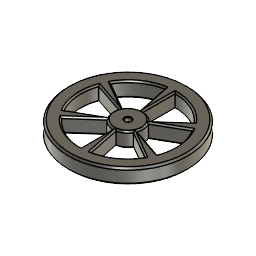
main_build (Autodesk Fusion 360 archive; units mm, degrees)
design "80x10 wheel"
Autodesk Fusion 360 part; units mm, degrees
sketch "Sketch1" plane through (0, 0, 0) normal (0, 0, 1) x (1, 0, 0)
  circle A0 centre (0, 0) radius 40
  dimension "d1" = 80
  constraint coincident A0.centre origin
  measures "d1" diameter of A0
extrude "Extrude1" add sketch "Sketch1" along normal blind 10
chamfer "Chamfer1" distance 1.2 angle 45 2 edges at (-37.2931, -14.4646, 10) (-37.2931, -14.4646, 0)
sketch "Sketch2" plane through (0, 0, 10) normal (0, 0, 1) x (-1, 0, 0)
  circle A0 centre (0, 0) radius 38.8
  circle A1 centre (0, 0) radius 1.5
  dimension "d5" = 3
  constraint coincident A0.centre A1.centre
  measures "d5" diameter of A1
extrude "Extrude2" cut sketch "Sketch2" against normal blind 25 contours A1
sketch "Sketch3" plane through (0, 0, 10) normal (0, 0, 1) x (-1, 0, 0)
  circle A0 centre (0, 0) radius 1.5
  circle A1 centre (0, 0) radius 38.8
  circle A2 centre (0, 0) radius 31.5
  circle A3 centre (0, 0) radius 10
  line L0 (0, -10) -> (0, -31.5)
  line L1 (-7.6037, -6.4949) -> (-23.6999, -20.75)
  dimension "d8" = 63
  dimension "d9" = 20
  constraint coincident A0.centre A1.centre
  constraint coincident A3 L0.start
  constraint coincident A2 L0.end
  constraint vertical L0
  constraint coincident A3 L1.start
  constraint coincident A2 L1.end
  measures "d8" diameter of A2
  measures "d9" diameter of A3
extrude "Extrude3" cut sketch "Sketch3" against normal blind 25 contours A2 A3 L0 L1 picked at (-16.9397, -17.3876)
chamfer "Chamfer2" distance 1 angle 45 6 edges at (13.012, 28.6869, 10) (15.6518, 13.6224, 10) (15.6518, 13.6224, 0) (0, 20.75, 10) (13.012, 28.6869, 0) (0, 20.75, 0)
pattern_circular "C-Pattern1" count 6 over 360 about axis through (0, 0, 1.75) along (0, 0, 1) of "Extrude3", "Chamfer2"
chamfer "Chamfer3" distance 1 angle 45 2 edges at (9.3233, 3.6162, 10) (7.7933, -6.2661, 0)
move_face "OffsetFaces1" offset -0.5 1 faces at (-1.4925, 0.1494, 6.6667)
chamfer "Chamfer4" distance 0.4 angle 45 1 edges at (1.8647, 0.7232, 0)
chamfer "Chamfer5" distance 0.4 angle 45 1 edges at (1.8647, -0.7232, 10)

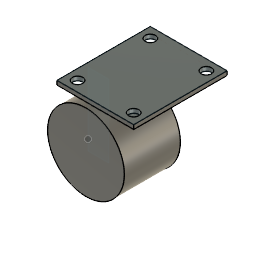
design "trolley_wheel"
Autodesk Fusion 360 part; units mm, degrees
sketch "Sketch1" plane through (0, 0, 0) normal (0, 0, 1) x (1, 0, 0)
  line L0 (0, 0) -> (37, 0)
  line L1 (37, 0) -> (37, 45)
  line L2 (37, 45) -> (0, 45)
  line L3 (0, 45) -> (0, 0)
  dimension "d1" = 37
  dimension "d2" = 45
  constraint horizontal L0
  constraint vertical L1
  constraint horizontal L2
  constraint vertical L3
  constraint coincident L0.start L3.end
  measures "d1" distance of L0.start L0.end
  measures "d2" distance of L0.start L2.end
extrude "Extrude1" add sketch "Sketch1" along normal blind 2
sketch "Sketch2" plane through (0, 0, 2) normal (0, 0, 1) x (-1, 0, 0)
  line L0 (0, -45) -> (0, 0)
  line L1 (0, 0) -> (-37, 0)
  line L2 (-37, 0) -> (-37, -45)
  line L3 (-37, -45) -> (0, -45)
sketch "Sketch3" plane through (0, 0, 2) normal (0, 0, 1) x (-1, 0, 0)
sketch "Sketch4" plane through (0, 0, 2) normal (0, 0, 1) x (-1, 0, 0)
  point P0 (-5, -40)
hole "Hole1" at (5, 40, 2) direction (0, 0, -1) diameter 5 depth 15 tip angle 180
ref_plane "WorkPlane1" through (18.5, 22.5, 1) normal (1, 0, 0) x (0, 1, 0)
ref_plane "WorkPlane2" through (18.5, 22.5, 1) normal (0, -1, 0) x (1, 0, 0)
mirror "Mirror1" about plane through (18.5, 22.5, 1) normal (1, 0, 0) of "Hole1"
mirror "Mirror2" about plane through (18.5, 22.5, 1) normal (0, -1, 0) of "Hole1", "Mirror1"
sketch "Sketch5" plane through (0, 0, 0) normal (0, 0, -1) x (1, 0, 0)
  circle A0 centre (32, -5) radius 2.5
  circle A1 centre (5, -5) radius 2.5
  circle A2 centre (32, -40) radius 2.5
  circle A3 centre (5, -40) radius 2.5
  line L0 (0, 0) -> (0, -45)
  line L1 (0, -45) -> (37, -45)
  line L2 (37, -45) -> (37, 0)
  line L3 (37, 0) -> (0, 0)
  line L4 (0, -15) -> (10, -15)
  line L5 (10, -15) -> (10, -25)
  line L6 (10, -25) -> (0, -25)
  line L7 (0, -25) -> (0, -15)
  constraint horizontal L4
  constraint vertical L5
  constraint horizontal L6
  constraint vertical L7
  constraint coincident L0 L4.start
extrude "Extrude2" add sketch "Sketch5" along normal blind 35 contours L0 L4 L5 L6 L7
sketch "Sketch6" plane through (0, 15, 0) normal (0, -1, 0) x (1, 0, 0)
  line L0 (10, 0) -> (0, 0)
  line L1 (0, 0) -> (0, -35)
  line L2 (0, -35) -> (10, -35)
  line L3 (10, -35) -> (10, 0)
  point P0 (0, -30)
  constraint coincident L1 P0
sketch "Sketch7" plane through (0, 15, 0) normal (0, -1, 0) x (1, 0, 0)
sketch "Sketch8" plane through (0, 15, 0) normal (0, -1, 0) x (1, 0, 0)
  circle A0 centre (5, -30) radius 18.5
  dimension "d14" = 37
  measures "d14" diameter of A0
extrude "Extrude3" add sketch "Sketch8" against normal blind 16
extrude "Extrude4" add 1 faces at (3.6278, 31, -23.9879) along direction (0, -1, 0) blind 22
extrude "Extrude5" add 1 faces at (5, 25, -3.8333) along direction (0, 1, 0) blind 5
extrude "Extrude6" add 1 faces at (3.6278, 31, -23.9879) along direction (0, 1, 0) blind 5
